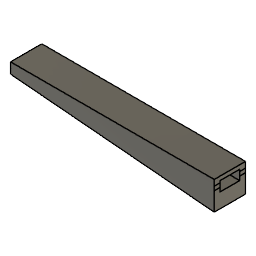
BoTech.StarClock.LedStripMountingPlate (Autodesk Fusion 360 design; units mm, degrees)
Autodesk Fusion 360 part; units mm, degrees
sketch "Skizze1" plane through (0, 0, 0) normal (0, 1, 0) x (1, 0, 0)
  line L0 (-104, -11.5) -> (-104, -9.5)
  line L1 (0, -9.5) -> (0, -11.5)
  line L2 (-104, -9.5) -> (0, -9.5)
  line L3 (0, -9.5) -> (0, 0)
  line L4 (-104, -9.5) -> (-104, -9.05)
  line L5 (0, 0) -> (-104, -9.05)
  line L6 (0, -11.5) -> (-104, -11.5)
  line L7 (-104, -11.5) -> (-104, -14.5)
  line L8 (-104, -14.5) -> (0, -14.5)
  line L9 (0, -14.5) -> (0, -11.5)
  dimension "d2" = 2
  dimension "d3" = 104
  dimension "d4" = 3
  dimension "d5" = 2
  constraint perpendicular L1 L2
  constraint perpendicular L2 L4
  constraint perpendicular L2 L3
  constraint horizontal L6
  constraint vertical L7
  constraint horizontal L8
  constraint vertical L9
  measures "d2" distance of L1.start L1.end
  measures "d3" distance of L1.end L0.start
  measures "d4" distance of L1.end L8.end
  measures "d5" distance of L0.end L0.start
extrude "Extrusion1" add sketch "Skizze1" along normal blind 16
sketch "Skizze2" plane through (-104, 0, -0.0001) normal (-1, 0, -0.000001) x (0, -1, 0)
  line L0 (0, 9.5001) -> (0, 11.5001)
  line L1 (0, 11.5001) -> (-16, 11.5001)
  line L2 (-16, 11.5001) -> (-16, 9.5001)
  line L3 (-16, 9.5001) -> (0, 9.5001)
  line L4 (-13, 14.5) -> (-13, 12.5)
  line L5 (-13, 12.5) -> (-16, 12.5)
  line L6 (-13, 12.5) -> (-3, 12.5)
  line L7 (-3, 12.5) -> (0, 12.5)
  line L8 (0, 12.5) -> (-3, 12.5)
  line L9 (-3, 12.5) -> (-3, 7.5)
  line L10 (-3, 7.5) -> (-13, 7.5)
  line L11 (-13, 7.5) -> (-13, 12.5)
  dimension "d11" = 3
  dimension "d12" = 10
  dimension "d13" = 3
  dimension "d14" = 5
  constraint vertical L4
  constraint perpendicular L4 L5
  constraint perpendicular L4 L6
  constraint perpendicular L4 L7
  constraint perpendicular L3 L9
  constraint perpendicular L9 L10
  measures "d11" distance of L4.end L5.end
  measures "d12" distance of L4.end L6.end
  measures "d13" distance of L6.end L7.end
  measures "d14" distance of L6.end L9.end
extrude "Extrusion2" cut sketch "Skizze2" against normal blind 105.5 contours L3 L9 L10 L11 | L1 L3 L9 L11 | L1 L6 L9 L11
